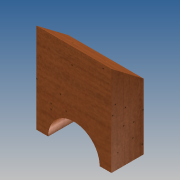
# Autodesk Inventor part: 2p4irsh
Saved by Autodesk Inventor 2014 SP1 (Build 180222100, 222)
## iProperties
Company: HERA Project
Created: 2013-12-04
Part Number: 2p4irsh
Material: Wood (Cherry)
Document SubType Name: Modeling
Designer: David DeBoer
Mass: 283.669 g
Surface Area: 501.887 cm^2
Volume: 567.338 cm^3
Density: 0.5 g/cm^3
Description: intermediate rim spar holder
Appearance: Cherry - Natural Low Gloss
Author: David DeBoer
Autodesk Inventor part; units mm, degrees
ref_plane "YZ Plane" through (0, 0, 0) normal (1, 0, 0) x (0, 1, 0)
ref_plane "XZ Plane" through (0, 0, 0) normal (0, 1, 0) x (-1, 0, 0)
ref_plane "XY Plane" through (0, 0, 0) normal (0, 0, 1) x (1, 0, 0)
sketch "Sketch1" plane through (0, 0, 0) normal (1, 0, 0) x (0, 1, 0)
  line L0 (0, 0) -> (106.68, 0)
  line L1 (0, 0) -> (0, -38.1)
  line L2 (106.68, 0) -> (77.7888, -38.1)
  line L3 (106.68, 0) -> (170.6921, 0) construction
  line L4 (0, -38.1) -> (77.7888, -38.1)
  dimension "d2" = 106.68
  dimension "d4" = 38.1
  dimension "d26" = 127.173
  constraints: 10 end point, 2 horizontal, 1 parallel, 1 perpendicular
  measures "d2" distance of L0.start L0.end
  measures "d4" distance of L0.start L1.end
  measures "d26" angle of L2 L3
extrude "Extrusion1" add sketch "Sketch1" along normal blind 88.9
sketch "Sketch2" plane through (0, 0, 0) normal (0, 0, 1) x (1, 0, 0)
  line L0 (0, 0) -> (88.9, 0) projected
  circle A0 centre (44.45, 0) radius 30.48
  dimension "d8" = 60.96
  constraints: 1 centre point, 1 midpoint
  measures "d8" diameter of A0
extrude "Extrusion2" cut sketch "Sketch2" against normal blind 88.9
sketch "Sketch4" plane through (0, 106.68, 0) normal (0, 0.7968147, -0.6042237) x (1, 0, 0)
  line L0 (88.9, 47.8154) -> (88.9, 0) projected
  line L1 (0, 47.8154) -> (88.9, 47.8154) projected
  circle A0 centre (63.5, 23.8532) radius 2.921
  line L2 (0, 0) -> (0, 47.8154) projected
  point P0 (0, 64.4586)
  point P1 (25.4, 23.8532)
  dimension "d27" = 25.4
  dimension "d30" = 38.1
  dimension "d42" = 25.4
  constraints: 1 centre point, 1 horizontal, 1 other
  measures "d27" distance from line of L0 A0.centre
  measures "d30" distance of A0.centre point (25.4, 23.853)
  measures "d42" distance from line of L2 point (25.4, 23.853)
hole "Hole2" at (25.4, 92.2673, -19.0066) at (63.5, 92.2673, -19.0066) direction (0, -0.7968147, 0.6042237) diameter 3.175 depth 25.4 tip angle 118
body "Solid1"
